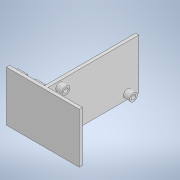
# Autodesk Inventor part: prototype_5_testPart1
Saved by Autodesk Inventor 2022 (Build 260153000, 153)
## iProperties
Created: 2022-06-10
Part Number: prototype_5_testPart1
Material: Generic
Document SubType Name: Modeling
Designer: tecware
Density: 1 g/cm^3
Appearance: Default
Author: tecware
## iProperties of the stored document prototype_5_testPart1_3DPrint.ipt
Created: 2022-06-10
Part Number: prototype_5_testPart1_3DPrint
Material: Generic
Document SubType Name: Modeling
Designer: tecware
Density: 1 g/cm^3
Appearance: Default
Author: tecware
Autodesk Inventor part; units mm, degrees
ref_plane "YZ Plane" through (0, 0, 0) normal (1, 0, 0) x (0, 1, 0)
ref_plane "XZ Plane" through (0, 0, 0) normal (0, 1, 0) x (-1, 0, 0)
ref_plane "XY Plane" through (0, 0, 0) normal (0, 0, 1) x (1, 0, 0)
sketch "Sketch1" plane through (0, 0, 0) normal (0, 0, 1) x (1, 0, 0)
  line L0 (8.8, 13.8) -> (-8.8, 13.8)
  line L1 (-8.8, 13.8) -> (-8.8, -13.8)
  line L2 (-8.8, -13.8) -> (8.8, -13.8)
  line L3 (8.8, -13.8) -> (8.8, 13.8)
  line L4 (8.8, 13.8) -> (-8.8, -13.8) construction
  line L5 (-8.8, 13.8) -> (8.8, -13.8) construction
  line L6 (8.8, 0) -> (-8.8, 0) construction
  line L7 (2.5, -13.8) -> (-2.5, -13.8)
  line L8 (-2.5, -8.8) -> (2.5, -8.8)
  line L9 (2.5, -8.8) -> (2.5, -13.8)
  line L10 (2.5, -13.8) -> (-2.5, -8.8) construction
  line L11 (-2.5, -13.8) -> (2.5, -8.8) construction
  line L12 (-2.5, -8.8) -> (-2.5, -13.8)
  line L13 (3.8, -2.5) -> (8.8, -2.5)
  line L14 (3.8, 8.8) -> (-3.8, 8.8)
  line L15 (-3.8, 8.8) -> (-3.8, -8.8)
  line L16 (-3.8, -8.8) -> (3.8, -8.8)
  line L17 (3.8, -8.8) -> (3.8, 8.8)
  line L18 (3.8, 8.8) -> (-3.8, -8.8) construction
  line L19 (-3.8, 8.8) -> (3.8, -8.8) construction
  line L20 (-3.8, -2.5) -> (-8.8, -2.5)
  line L21 (2.5, 13.8) -> (-2.5, 13.8)
  line L22 (-2.5, 8.8) -> (2.5, 8.8)
  line L23 (2.5, 8.8) -> (2.5, 13.8)
  line L24 (2.5, 13.8) -> (-2.5, 8.8) construction
  line L25 (-2.5, 13.8) -> (2.5, 8.8) construction
  line L26 (-2.5, 8.8) -> (-2.5, 13.8)
  line L27 (3.8, 2.5) -> (8.8, 2.5)
  line L28 (-3.8, 2.5) -> (-8.8, 2.5)
  point P0 (0, 0)
  dimension "d0" = 17.6
  dimension "d1" = 27.6
  dimension "d5" = 5
  dimension "d7" = 7.6
  dimension "d8" = 17.6
  constraints: 58 end point, 8 symmetric about line, 6 midpoint, 2 point on line
  measures "d0" distance of L2.end L1.end
  measures "d1" distance of L1.end L0.end
  measures "d5" distance of L13.end L13.start
  measures "d7" distance of L16.end L15.end
  measures "d8" distance of L15.end L14.end
extrude "Extrusion1" add sketch "Sketch1" against normal blind 3 contours L3 L27 L17 L14 L23 L0 | L26 L14 L15 L28 L1 L0 | L3 L2 L9 L16 L17 L13 | L20 L15 L16 L12 L2 L1
sketch "Sketch2" plane through (0, 0, 0) normal (0, 0, 1) x (1, 0, 0)
  line L0 (11, 16) -> (-11, 16)
  line L1 (-11, 16) -> (-11, -16)
  line L2 (-11, -16) -> (11, -16)
  line L3 (11, -16) -> (11, 16)
  line L4 (11, 16) -> (-11, -16) construction
  line L5 (-11, 16) -> (11, -16) construction
  line L6 (11, 16) -> (11.4, 16)
  line L7 (11.4, 16) -> (11.4, -16)
  line L8 (11.4, -16) -> (11, -16)
  line L9 (11, -16) -> (11, 16)
  point P0 (0, 0)
  dimension "d11" = 22
  dimension "d12" = 32
  dimension "d18" = 0.4
  constraints: 20 end point, 2 midpoint
  measures "d11" distance of L2.end L1.end
  measures "d12" distance of L1.end L0.end
  measures "d18" distance of L7.end L8.end
extrude "Extrusion2" add sketch "Sketch2" along normal blind 2
sketch "Sketch3" plane through (11.4, -16, 0) normal (1, 0, 0) x (0, 0, -1)
  line L0 (-2, 32) -> (-2, 0) projected
  line L1 (-2, 0) -> (58, 0)
  line L2 (58, 0) -> (58, 32)
  line L3 (58, 32) -> (-2, 32)
  line L4 (-2, 32) -> (-2, 0)
  point P0 (0, 16)
  dimension "d15" = 60
  constraints: 8 end point
  measures "d15" distance of L3.end L2.end
extrude "Extrusion3" add sketch "Sketch3" along normal blind 2
sketch "Sketch5" plane through (11.4, -16, 0) normal (-1, 0, 0) x (0, 0, 1)
  line L0 (-2, 14.5) -> (0, 14.5)
  line L1 (0, 14.5) -> (0, 17.5)
  line L2 (0, 17.5) -> (-2, 17.5)
  line L3 (-2, 17.5) -> (-2, 14.5)
  point P0 (0, 16)
  point P1 (0, 16)
  dimension "d19" = 2
  dimension "d20" = 3
  constraints: 8 end point, 1 midpoint
  measures "d19" distance of L2.end L1.end
  measures "d20" distance of L1.end L0.end
extrude "Extrusion4" cut sketch "Sketch5" against normal up to surface (2 mm away)
sketch "Sketch6" plane through (13.4, -16, 0) normal (1, 0, 0) x (0, 0, -1)
  line L0 (0, 32) -> (0, 0) projected
  line L1 (-2, 32) -> (0, 32)
  line L2 (0, 32) -> (0, 0)
  line L3 (0, 0) -> (-2, 0)
  line L4 (-2, 0) -> (-2, 32)
  point P0 (0, 16)
  constraints: 8 end point
extrude "Extrusion5" add sketch "Sketch6" along normal blind 22
sketch "Sketch7" plane through (13.4, -16, 0) normal (1, 0, 0) x (0, 0, -1)
  circle A0 centre (50.5, 3.4) radius 2.5
  circle A1 centre (50.5, 3.4) radius 1.4
  circle A2 centre (7.5, 28.6) radius 2.5
  circle A3 centre (7.5, 28.6) radius 1.4
  line L0 (0, 0) -> (58, 0) projected
  line L1 (58, 0) -> (58, 32) projected
  line L2 (58, 32) -> (0, 32) projected
  line L3 (0, 0) -> (0, 32) projected
  point P0 (0, 16)
  dimension "d25" = 5
  dimension "d26" = 2.8
  dimension "d27" = 5
  dimension "d28" = 2.8
  dimension "d29" = 3.4
  dimension "d30" = 7.5
  dimension "d31" = 3.4
  dimension "d32" = 7.5
  constraints: 4 centre point, 2 coincident
  measures "d25" diameter of A0
  measures "d26" diameter of A1
  measures "d27" diameter of A2
  measures "d28" diameter of A3
  measures "d29" distance from line of L0 A0.centre
  measures "d30" distance from line of L1 A0.centre
  measures "d31" distance from line of L2 A2.centre
  measures "d32" distance from line of L3 A2.centre
extrude "Extrusion6" add sketch "Sketch7" along normal blind 4 contours A0 | A2
body "Solid1"
